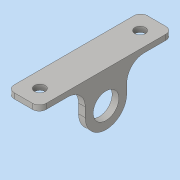
# Autodesk Inventor part: ToggleSwitchBracket
Saved by Autodesk Inventor 2016 (Build 200138000, 138)
## iProperties
Created: 2015-12-17
Part Number: ToggleSwitchBracket
Material: Generic
Document SubType Name: Modeling
Designer: rahuliyer
Density: 1 g/cm^3
Appearance: Default
Author: rahuliyer
Autodesk Inventor part; units mm, degrees
ref_plane "YZ Plane" through (0, 0, 0) normal (1, 0, 0) x (0, 1, 0)
ref_plane "XZ Plane" through (0, 0, 0) normal (0, 1, 0) x (-1, 0, 0)
ref_plane "XY Plane" through (0, 0, 0) normal (0, 0, 1) x (1, 0, 0)
sketch "Sketch1" plane through (0, 0, 0) normal (1, 0, 0) x (0, 1, 0)
  circle A0 centre (0, 0) radius 6.096
  arc A1 (0, 9.906) -> (0, -9.906) centre (0, 0) ccw
  line L0 (0, 9.906) -> (12.7, 9.906)
  line L1 (12.7, 9.906) -> (12.7, -9.906)
  line L2 (12.7, -9.906) -> (0, -9.906)
  arc A2 (0, -9.906) -> (0, 9.906) centre (0, 0) ccw construction
  dimension "d0" = 12.192
  dimension "d1" = 3.81
  dimension "d2" = 12.7
  constraints: 6 end point, 4 point on circle, 3 centre point, 2 horizontal, 1 coincident, 1 perpendicular, 1 tangent, 1 vertical alignment
  measures "d0" diameter of A0
  measures "d1" radial gap between concentric circles of A0 A1
  measures "d2" distance from line of point (0, 0) L1
extrude "Extrusion1" add sketch "Sketch1" along normal blind 3.175
sketch "Sketch3" plane through (0, 12.7, 9.906) normal (0, 1, 0) x (1, 0, 0)
  line L0 (-12.065, 41.656) -> (3.175, 41.656)
  line L1 (3.175, 41.656) -> (3.175, -21.844)
  line L2 (3.175, -21.844) -> (-12.065, -21.844)
  line L3 (-12.065, -21.844) -> (-12.065, 41.656)
  line L4 (3.175, 19.812) -> (3.175, 0) projected
  circle A0 centre (-4.445, 33.782) radius 2.5527
  circle A1 centre (-4.445, -13.97) radius 2.5527
  line L5 (-12.065, 9.906) -> (3.175, 9.906) construction
  point P0 (0, 9.906)
  dimension "d6" = 63.5
  dimension "d7" = 15.24
  dimension "d8" = 5.1054
  dimension "d9" = 47.752
  dimension "d10" = 7.62
  constraints: 10 end point, 3 midpoint, 2 centre point, 2 horizontal, 2 parallel, 1 collinear, 1 equal radius, 1 perpendicular, 1 symmetric about line
  measures "d6" distance of L2.end L0.start
  measures "d7" distance between parallel lines of L1 L3
  measures "d8" diameter of A1
  measures "d9" distance of A1.centre A0.centre
  measures "d10" distance from line of L1 A0.centre
extrude "Extrusion2" add sketch "Sketch3" along normal blind 2.54
fillet "Fillet1" radius 8.255 2 edges at (1.5875, 12.7, -9.906) (1.5875, 12.7, 9.906)
fillet "Fillet2" radius 1.27 1 edges at (0, 12.7, 0)
fillet "Fillet3" radius 3.175 4 edges at (-12.065, 13.97, -31.75) (3.175, 13.97, -31.75) (3.175, 13.97, 31.75) (-12.065, 13.97, 31.75)
body "Solid1"
